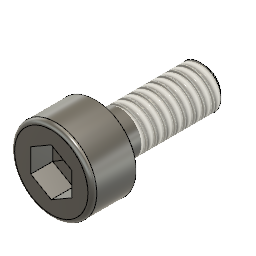
oscillating_design v15 (Autodesk Fusion 360 archive; units mm, degrees)
design "Broached Hexagon Socket Head Cap Screw ASME B18.3.1M - M1.6x0.35 x 4 Steel Grade 2 Plain"
description: Broached Hexagon Socket Head Cap Screw ASME B18.3.1M - M1.6x0.35 x 4
part number: BSHCS ASME B18.3.1M - M1.6x0.35 x 4 Steel Grade 2 Plain
Autodesk Fusion 360 part; units mm, degrees
sketch "Sketch1" plane through (0, 0, 0) normal (0, 1, 0) x (1, 0, 0)
  line L0 (-0.8, 0) -> (-0.8, 4)
  line L1 (-0.8, 4) -> (0, 4)
  line L2 (0, 4) -> (0, -1.6)
  line L3 (-0.8, 0) -> (-1.5, 0)
  line L4 (-1.5, 0) -> (-1.5, -1.6)
  line L5 (-1.5, -1.6) -> (0, -1.6)
  dimension "d9" = 1.6
  dimension "d66" = 3
  dimension "d101" = 4
  dimension "d102" = 1.6
  constraint perpendicular L0 L1
  constraint collinear origin L1.end L2.end
  constraint perpendicular L0 L3
  constraint coincident origin L3
  constraint vertical L0
  constraint vertical L2
  constraint parallel L2 L4
  constraint coincident L2 L5.end
  constraint perpendicular L2 L5
  measures "d101" distance of origin L1
  measures "d102" distance of L3.end L5
revolve "Revolve1" add sketch "Sketch1" angle 360 about axis through (0, 0, -4) along (0, 0, 1)
ref_plane "WorkPlane1" through (0, 0, 1.6) normal (0, 0, 1) x (1, 0, 0)
sketch "Sketch6" plane through (0, 0, 1.6) normal (0, 0, 1) x (1, 0, 0)
  line L0 (-0.75, 0) -> (0.75, 0) construction
  line L1 (0, 0) -> (-0.75, 0.433)
  line L2 (-0.75, -0.433) -> (-0.75, 0.433)
  line L3 (-0.75, -0.433) -> (0, 0)
  dimension "d100" = 150
  dimension "d103" = 1.5
  constraint horizontal L0
  constraint midpoint L1.start L0
  constraint coincident L1.start L3.end
  constraint perpendicular L0 L2
  constraint midpoint L0.start L2
  constraint coincident L1.end L2.end
  measures "d100" angle of L0 L1
  measures "d103" distance of L0.end L2
extrude "Extrude1" cut sketch "Sketch6" against normal blind 0.8
pattern_circular "C-Pattern1" count 6 over 360 about axis through (0, 0, 1.75) along (0, 0, 1) of "Extrude1"
extrude "Extrude2" cut 1 faces at (0, 0.2887, 0.8) along direction (0, 0, -1) blind 0.8 draft -85
thread "Thread2" "ANSI Metric M Profile 1.6 M1.6x0.35 4g6g" major diameter 1.5385 minor diameter 1.15 pitch 0.35 angle 60 resizes the face on face at (-0.796, 0.0797, -2.6667) from (0, 0, -0.9147) to (0, 0, -4)
fillet "Fillet4" radius 0.16 1 edges at (-1.3985, 0.5424, 1.6)
sketch "Sketch7" plane through (0, 0, 0) normal (0, 1, 0) x (1, 0, 0)
  line L0 (-0.816, 4) -> (-0.816, 3.7853)
  line L1 (-0.816, 3.7853) -> (-0.5853, 4)
  line L2 (0, 4) -> (0, -1.6)
  line L3 (-0.816, 4) -> (0, 4)
  dimension "d104" = 0.5853
  dimension "d105" = 0.816
  dimension "d106" = 0.2147
  constraint coincident L2.start L3.end
  constraint perpendicular L2 L3
  constraint coincident L1.end L3
  constraint perpendicular L0 L3
  measures "d104" distance of L1.end L2
  measures "d105" distance of L0 L2.start
  measures "d106" distance of L0.end L3
revolve "Revolve3" cut sketch "Sketch7" angle 360 about axis through (0, 0, 1.75) along (0, 0, 1)
equation "d9 = adsk_nomdia"
equation "adsk_nomlen = 4.00 mm"
equation "adsk_headh = 1.60 mm"
equation "adsk_headdia = 3.00 mm"
equation "adsk_nomdia = 1.60 mm"
equation "adsk_philwidth = 1.50 mm"
equation "d31 = -adsk_phildepth"
equation "adsk_phildepth = 0.80 mm"
equation "d66 = adsk_headdia"
equation "d71 = adsk_headh"
equation "d76 = -adsk_phildepth"
equation "adsk_thrlen = 3.0852925 mm"
equation "d84 = adsk_thrlen"
equation "d86 = adsk_nomdia * 0.1"
equation "adsk_startlen = 0.2147075 mm"
equation "adsk_endpointdia = 1.170585 mm"
equation "d101 = adsk_nomlen"
equation "d102 = adsk_headh"
equation "d103 = adsk_philwidth"
equation "d104 = adsk_endpointdia / 2"
equation "d105 = adsk_nomdia * 0.51"
equation "d106 = adsk_startlen"

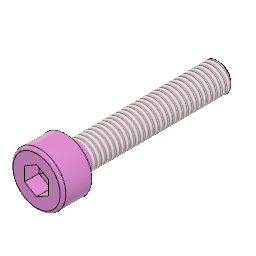
design "Broached Hexagon Socket Head Cap Screw ASME B18.3.1M - M3x0.5 x 16 Steel Grade 2 Plain"
description: Broached Hexagon Socket Head Cap Screw ASME B18.3.1M - M3x0.5 x 16
part number: BSHCS ASME B18.3.1M - M3x0.5 x 16 Steel Grade 2 Plain
Autodesk Fusion 360 part; units mm, degrees
sketch "Sketch1" plane through (0, 0, 0) normal (0, 1, 0) x (1, 0, 0)
  line L0 (-1.5, 0) -> (-1.5, 16)
  line L1 (-1.5, 16) -> (0, 16)
  line L2 (0, 16) -> (0, -3)
  line L3 (-1.5, 0) -> (-2.75, 0)
  line L4 (-2.75, 0) -> (-2.75, -3)
  line L5 (-2.75, -3) -> (0, -3)
  dimension "d9" = 3
  dimension "d66" = 5.5
  dimension "d101" = 16
  dimension "d102" = 3
  constraint perpendicular L0 L1
  constraint collinear origin L1.end L2.end
  constraint perpendicular L0 L3
  constraint coincident origin L3
  constraint vertical L0
  constraint vertical L2
  constraint parallel L2 L4
  constraint coincident L2 L5.end
  constraint perpendicular L2 L5
  measures "d101" distance of origin L1
  measures "d102" distance of L3.end L5
revolve "Revolve1" add sketch "Sketch1" angle 360 about axis through (0, 0, -16) along (0, 0, 1)
ref_plane "WorkPlane1" through (0, 0, 3) normal (0, 0, 1) x (1, 0, 0)
sketch "Sketch6" plane through (0, 0, 3) normal (0, 0, 1) x (1, 0, 0)
  line L0 (-1.25, 0) -> (1.25, 0) construction
  line L1 (0, 0) -> (-1.25, 0.7217)
  line L2 (-1.25, -0.7217) -> (-1.25, 0.7217)
  line L3 (-1.25, -0.7217) -> (0, 0)
  dimension "d100" = 150
  dimension "d103" = 2.5
  constraint horizontal L0
  constraint midpoint L1.start L0
  constraint coincident L1.start L3.end
  constraint perpendicular L0 L2
  constraint midpoint L0.start L2
  constraint coincident L1.end L2.end
  measures "d100" angle of L0 L1
  measures "d103" distance of L0.end L2
extrude "Extrude1" cut sketch "Sketch6" against normal blind 1.5
pattern_circular "C-Pattern1" count 6 over 360 about axis through (0, 0, 1.75) along (0, 0, 1) of "Extrude1"
extrude "Extrude2" cut 1 faces at (0, -0.4811, 1.5) along direction (0, 0, -1) blind 1.5 draft -85
thread "Thread2" "ANSI Metric M Profile 3.0 M3x0.5 4g6g" major diameter 2.927 minor diameter 2.369 pitch 0.5 angle 60 resizes the face on face at (-1.4925, 0.1494, -10.6667) from (0, 0, -1.3067) to (0, 0, -16)
fillet "Fillet4" radius 0.3 1 edges at (-2.5639, 0.9944, 3)
sketch "Sketch7" plane through (0, 0, 0) normal (0, 1, 0) x (1, 0, 0)
  line L0 (-1.53, 16) -> (-1.53, 15.6933)
  line L1 (-1.53, 15.6933) -> (-1.1933, 16)
  line L2 (0, 16) -> (0, -3)
  line L3 (-1.53, 16) -> (0, 16)
  dimension "d104" = 1.1933
  dimension "d105" = 1.53
  dimension "d106" = 0.3067
  constraint coincident L2.start L3.end
  constraint perpendicular L2 L3
  constraint coincident L1.end L3
  constraint perpendicular L0 L3
  measures "d104" distance of L1.end L2
  measures "d105" distance of L0 L2.start
  measures "d106" distance of L0.end L3
revolve "Revolve3" cut sketch "Sketch7" angle 360 about axis through (0, 0, 1.75) along (0, 0, 1)
equation "d9 = adsk_nomdia"
equation "adsk_nomlen = 16.00 mm"
equation "adsk_headh = 3.00 mm"
equation "adsk_headdia = 5.50 mm"
equation "adsk_nomdia = 3.00 mm"
equation "adsk_philwidth = 2.50 mm"
equation "d31 = -adsk_phildepth"
equation "adsk_phildepth = 1.50 mm"
equation "d66 = adsk_headdia"
equation "d71 = adsk_headh"
equation "d76 = -adsk_phildepth"
equation "adsk_thrlen = 14.693275 mm"
equation "d84 = adsk_thrlen"
equation "d86 = adsk_nomdia * 0.1"
equation "adsk_startlen = 0.306725 mm"
equation "adsk_endpointdia = 2.38655 mm"
equation "d101 = adsk_nomlen"
equation "d102 = adsk_headh"
equation "d103 = adsk_philwidth"
equation "d104 = adsk_endpointdia / 2"
equation "d105 = adsk_nomdia * 0.51"
equation "d106 = adsk_startlen"

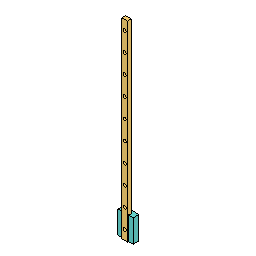
design "guide_rail"
Autodesk Fusion 360 part; units mm, degrees
sketch "Sketch1" plane through (0, 0, 0) normal (0, 1, 0) x (1, 0, 0)
  line L0 (0, 0) -> (8, 0)
  line L1 (8, 0) -> (8, -3)
  line L2 (8, -3) -> (5.5, -3)
  line L3 (0, 0) -> (0, -3)
  line L4 (0, -3) -> (2.5, -3)
  line L5 (2.5, -3) -> (2.5, -2)
  line L6 (2.5, -2) -> (5.5, -2)
  line L7 (5.5, -3) -> (5.5, -2)
  line L8 (2.5, -2) -> (2.5, -4)
  line L9 (2.5, -4) -> (5.5, -4)
  line L10 (5.5, -4) -> (5.5, -2)
  dimension "d1" = 8
  dimension "d2" = 3
  dimension "d3" = 2.5
  dimension "d4" = 3
  dimension "d5" = 2.5
  dimension "d6" = 1
  dimension "d7" = 2
  dimension "d8" = 3
  constraint coincident L0.start L3.start
  constraint horizontal L0
  constraint perpendicular L0 L1
  constraint perpendicular L1 L2
  constraint perpendicular L0 L3
  constraint perpendicular L3 L4
  constraint perpendicular L0 L5
  constraint perpendicular L5 L6
  constraint perpendicular L6 L7
  constraint perpendicular L6 L8
  constraint perpendicular L8 L9
  measures "d1" distance of L0.start L0.end
  measures "d2" distance of L0.end L1.end
  measures "d3" distance of L1.end L2.end
  measures "d4" distance of L0.start L3.end
  measures "d5" distance of L3.end L4.end
  measures "d6" distance of L4.end L5.end
  measures "d7" distance of L5.end L8.end
  measures "d8" distance of L8.end L9.end
extrude "Extrude1" add sketch "Sketch1" along normal mid plane 12 contours L0 L1 L2 L3 L4 L5 L6 L7 L8 L10 makes body 1
extrude "Extrude2" add sketch "Sketch1" along normal mid plane 100 separate body contours L5 L6 L7 L8 L9 L10 makes body 2
sketch "Sketch2" plane through (0, 0, 0) normal (0, 0, -1) x (-1, 0, 0)
  line L0 (0, -6) -> (0, 6)
  line L1 (0, 6) -> (-8, 6)
  line L2 (-8, 6) -> (-8, -6)
  line L3 (-8, -6) -> (0, -6)
  line L4 (-4, -6) -> (-4, 6)
  circle A0 centre (-4, -1.75) radius 0.8
  circle A1 centre (-4, 1.75) radius 0.8
  line L5 (-4, -0.95) -> (-4, 0.95) construction
  point P0 (-4, 0)
  dimension "d14" = 1.6
  dimension "d15" = 1.6
  dimension "d16" = 3.5
  constraint midpoint L3 L4.start
  constraint midpoint L1 L4.end
  constraint coincident L4 A0.centre
  constraint coincident L4 A1.centre
  constraint coincident L4 L5.start
  constraint coincident A0 L5.start
  constraint coincident L4 L5.end
  constraint coincident A1 L5.end
  constraint midpoint L5 P0
  measures "d14" diameter of A0
  measures "d15" diameter of A1
  measures "d16" distance of A0.centre A1.centre
extrude "Extrude3" cut sketch "Sketch2" against normal blind 1.3 contours L4 A0 | L4 A0 | L4 A1 | L4 A1 bodies 2 1
sketch "Sketch3" plane through (0, 0, 2) normal (0, 0, -1) x (-1, 0, 0)
  line L0 (-2.5, -50) -> (-2.5, 50)
  line L1 (-2.5, 50) -> (-5.5, 50)
  line L2 (-5.5, 50) -> (-5.5, -50)
  line L3 (-5.5, -50) -> (-2.5, -50)
  circle A0 centre (-4, -45) radius 0.8
  circle A1 centre (-4, -35) radius 0.8
  circle A2 centre (-4, -25) radius 0.8
  circle A3 centre (-4, -15) radius 0.8
  circle A4 centre (-4, -5) radius 0.8
  circle A5 centre (-4, 5) radius 0.8
  circle A6 centre (-4, 15) radius 0.8
  circle A7 centre (-4, 25) radius 0.8
  circle A8 centre (-4, 35) radius 0.8
  circle A9 centre (-4, 45) radius 0.8
  dimension "d19" = 1.6
  dimension "d20" = 5
  dimension "d38" = 0
  dimension "d39" = 10
  measures "d19" diameter of A0
  measures "d20" distance of L3 A0.centre
extrude "Extrude4" cut sketch "Sketch3" against normal blind 11.812 contours A0 | A1 | A2 | A3 | A4 | A5 | A6 | A7 | A8 | A9 bodies 2
copy_body "Body->Comp1" bodies 2 removing the originals makes body 3 in component "rail"
copy_body "Body->Comp2" bodies 1 removing the originals makes body 4 in component "cart"
component "rail" placed x (1, 0, 0) y (0, 1, 0) z (0, 0, 1) at (0, 0, 0)
component "cart" placed x (-1, 0, 0) y (0, -1, 0) z (0, 0, 1) at (8, -44, 0.5)
equation "rail_length = 100 mm"
equation "d12 = rail_length / 2"
named bodies: "cart", "rail"

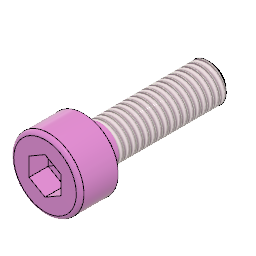
design "Broached Hexagon Socket Head Cap Screw ASME B18.3.1M - M3x0.5 x 10 Steel Grade 2 Plain"
description: Broached Hexagon Socket Head Cap Screw ASME B18.3.1M - M3x0.5 x 10
part number: BSHCS ASME B18.3.1M - M3x0.5 x 10 Steel Grade 2 Plain
Autodesk Fusion 360 part; units mm, degrees
sketch "Sketch1" plane through (0, 0, 0) normal (0, 1, 0) x (1, 0, 0)
  line L0 (-1.5, 0) -> (-1.5, 10)
  line L1 (-1.5, 10) -> (0, 10)
  line L2 (0, 10) -> (0, -3)
  line L3 (-1.5, 0) -> (-2.75, 0)
  line L4 (-2.75, 0) -> (-2.75, -3)
  line L5 (-2.75, -3) -> (0, -3)
  dimension "d9" = 3
  dimension "d66" = 5.5
  dimension "d101" = 10
  dimension "d102" = 3
  constraint perpendicular L0 L1
  constraint collinear origin L1.end L2.end
  constraint perpendicular L0 L3
  constraint coincident origin L3
  constraint vertical L0
  constraint vertical L2
  constraint parallel L2 L4
  constraint coincident L2 L5.end
  constraint perpendicular L2 L5
  measures "d101" distance of origin L1
  measures "d102" distance of L3.end L5
revolve "Revolve1" add sketch "Sketch1" angle 360 about axis through (0, 0, -10) along (0, 0, 1)
ref_plane "WorkPlane1" through (0, 0, 3) normal (0, 0, 1) x (1, 0, 0)
sketch "Sketch6" plane through (0, 0, 3) normal (0, 0, 1) x (1, 0, 0)
  line L0 (-1.25, 0) -> (1.25, 0) construction
  line L1 (0, 0) -> (-1.25, 0.7217)
  line L2 (-1.25, -0.7217) -> (-1.25, 0.7217)
  line L3 (-1.25, -0.7217) -> (0, 0)
  dimension "d100" = 150
  dimension "d103" = 2.5
  constraint horizontal L0
  constraint midpoint L1.start L0
  constraint coincident L1.start L3.end
  constraint perpendicular L0 L2
  constraint midpoint L0.start L2
  constraint coincident L1.end L2.end
  measures "d100" angle of L0 L1
  measures "d103" distance of L0.end L2
extrude "Extrude1" cut sketch "Sketch6" against normal blind 1.5
pattern_circular "C-Pattern1" count 6 over 360 about axis through (0, 0, 1.75) along (0, 0, 1) of "Extrude1"
extrude "Extrude2" cut 1 faces at (0, -0.4811, 1.5) along direction (0, 0, -1) blind 1.5 draft -85
thread "Thread2" "ANSI Metric M Profile 3.0 M3x0.5 4g6g" major diameter 2.927 minor diameter 2.369 pitch 0.5 angle 60 resizes the face on face at (-1.4925, 0.1494, -6.6667) from (0, 0, -1.3067) to (0, 0, -10)
fillet "Fillet4" radius 0.3 1 edges at (-2.5639, 0.9944, 3)
sketch "Sketch7" plane through (0, 0, 0) normal (0, 1, 0) x (1, 0, 0)
  line L0 (-1.53, 10) -> (-1.53, 9.6933)
  line L1 (-1.53, 9.6933) -> (-1.1933, 10)
  line L2 (0, 10) -> (0, -3)
  line L3 (-1.53, 10) -> (0, 10)
  dimension "d104" = 1.1933
  dimension "d105" = 1.53
  dimension "d106" = 0.3067
  constraint coincident L2.start L3.end
  constraint perpendicular L2 L3
  constraint coincident L1.end L3
  constraint perpendicular L0 L3
  measures "d104" distance of L1.end L2
  measures "d105" distance of L0 L2.start
  measures "d106" distance of L0.end L3
revolve "Revolve3" cut sketch "Sketch7" angle 360 about axis through (0, 0, 1.75) along (0, 0, 1)
equation "d9 = adsk_nomdia"
equation "adsk_nomlen = 10.00 mm"
equation "adsk_headh = 3.00 mm"
equation "adsk_headdia = 5.50 mm"
equation "adsk_nomdia = 3.00 mm"
equation "adsk_philwidth = 2.50 mm"
equation "d31 = -adsk_phildepth"
equation "adsk_phildepth = 1.50 mm"
equation "d66 = adsk_headdia"
equation "d71 = adsk_headh"
equation "d76 = -adsk_phildepth"
equation "adsk_thrlen = 8.693275 mm"
equation "d84 = adsk_thrlen"
equation "d86 = adsk_nomdia * 0.1"
equation "adsk_startlen = 0.306725 mm"
equation "adsk_endpointdia = 2.38655 mm"
equation "d101 = adsk_nomlen"
equation "d102 = adsk_headh"
equation "d103 = adsk_philwidth"
equation "d104 = adsk_endpointdia / 2"
equation "d105 = adsk_nomdia * 0.51"
equation "d106 = adsk_startlen"

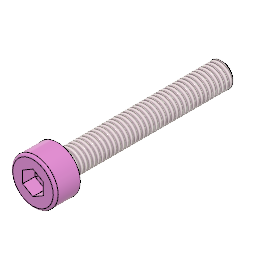
design "Broached Hexagon Socket Head Cap Screw ASME B18.3.1M - M3x0.5 x 20 Steel Grade 2 Plain"
description: Broached Hexagon Socket Head Cap Screw ASME B18.3.1M - M3x0.5 x 20
part number: BSHCS ASME B18.3.1M - M3x0.5 x 20 Steel Grade 2 Plain
Autodesk Fusion 360 part; units mm, degrees
sketch "Sketch1" plane through (0, 0, 0) normal (0, 1, 0) x (1, 0, 0)
  line L0 (-1.5, 0) -> (-1.5, 20)
  line L1 (-1.5, 20) -> (0, 20)
  line L2 (0, 20) -> (0, -3)
  line L3 (-1.5, 0) -> (-2.75, 0)
  line L4 (-2.75, 0) -> (-2.75, -3)
  line L5 (-2.75, -3) -> (0, -3)
  dimension "d9" = 3
  dimension "d66" = 5.5
  dimension "d101" = 20
  dimension "d102" = 3
  constraint perpendicular L0 L1
  constraint collinear origin L1.end L2.end
  constraint perpendicular L0 L3
  constraint coincident origin L3
  constraint vertical L0
  constraint vertical L2
  constraint parallel L2 L4
  constraint coincident L2 L5.end
  constraint perpendicular L2 L5
  measures "d101" distance of origin L1
  measures "d102" distance of L3.end L5
revolve "Revolve1" add sketch "Sketch1" angle 360 about axis through (0, 0, -20) along (0, 0, 1)
ref_plane "WorkPlane1" through (0, 0, 3) normal (0, 0, 1) x (1, 0, 0)
sketch "Sketch6" plane through (0, 0, 3) normal (0, 0, 1) x (1, 0, 0)
  line L0 (-1.25, 0) -> (1.25, 0) construction
  line L1 (0, 0) -> (-1.25, 0.7217)
  line L2 (-1.25, -0.7217) -> (-1.25, 0.7217)
  line L3 (-1.25, -0.7217) -> (0, 0)
  dimension "d100" = 150
  dimension "d103" = 2.5
  constraint horizontal L0
  constraint midpoint L1.start L0
  constraint coincident L1.start L3.end
  constraint perpendicular L0 L2
  constraint midpoint L0.start L2
  constraint coincident L1.end L2.end
  measures "d100" angle of L0 L1
  measures "d103" distance of L0.end L2
extrude "Extrude1" cut sketch "Sketch6" against normal blind 1.5
pattern_circular "C-Pattern1" count 6 over 360 about axis through (0, 0, 1.75) along (0, 0, 1) of "Extrude1"
extrude "Extrude2" cut 1 faces at (0, -0.4811, 1.5) along direction (0, 0, -1) blind 1.5 draft -85
thread "Thread2" "ANSI Metric M Profile 3.0 M3x0.5 4g6g" major diameter 2.927 minor diameter 2.369 pitch 0.5 angle 60 resizes the face on face at (-1.4925, 0.1494, -13.3333) from (0, 0, -0.9135) to (0, 0, -20)
fillet "Fillet4" radius 0.3 1 edges at (-2.5639, 0.9944, 3)
sketch "Sketch7" plane through (0, 0, 0) normal (0, 1, 0) x (1, 0, 0)
  line L0 (-1.53, 20) -> (-1.53, 19.6933)
  line L1 (-1.53, 19.6933) -> (-1.1933, 20)
  line L2 (0, 20) -> (0, -3)
  line L3 (-1.53, 20) -> (0, 20)
  dimension "d104" = 1.1933
  dimension "d105" = 1.53
  dimension "d106" = 0.3067
  constraint coincident L2.start L3.end
  constraint perpendicular L2 L3
  constraint coincident L1.end L3
  constraint perpendicular L0 L3
  measures "d104" distance of L1.end L2
  measures "d105" distance of L0 L2.start
  measures "d106" distance of L0.end L3
revolve "Revolve3" cut sketch "Sketch7" angle 360 about axis through (0, 0, 1.75) along (0, 0, 1)
equation "d9 = adsk_nomdia"
equation "adsk_nomlen = 20.00 mm"
equation "adsk_headh = 3.00 mm"
equation "adsk_headdia = 5.50 mm"
equation "adsk_nomdia = 3.00 mm"
equation "adsk_philwidth = 2.50 mm"
equation "d31 = -adsk_phildepth"
equation "adsk_phildepth = 1.50 mm"
equation "d66 = adsk_headdia"
equation "d71 = adsk_headh"
equation "d76 = -adsk_phildepth"
equation "adsk_thrlen = 19.08655 mm"
equation "d84 = adsk_thrlen"
equation "d86 = adsk_nomdia * 0.1"
equation "adsk_startlen = 0.306725 mm"
equation "adsk_endpointdia = 2.38655 mm"
equation "d101 = adsk_nomlen"
equation "d102 = adsk_headh"
equation "d103 = adsk_philwidth"
equation "d104 = adsk_endpointdia / 2"
equation "d105 = adsk_nomdia * 0.51"
equation "d106 = adsk_startlen"

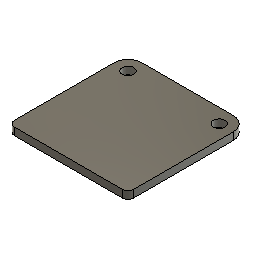
design "laser"
Autodesk Fusion 360 part; units mm, degrees
sketch "Sketch1" plane through (0, 0, 0) normal (0, 1, 0) x (1, 0, 0)
  line L0 (3, 0) -> (22.4, 0)
  line L1 (25.4, -3) -> (25.4, -24.13)
  line L2 (24.13, -25.4) -> (1.27, -25.4)
  line L3 (0, -24.13) -> (0, -3)
  line L4 (12.7, 0) -> (12.7, -25.4)
  circle A0 centre (3, -3) radius 1.25
  circle A1 centre (22.4, -3) radius 1.25
  arc A2 (3, 0) -> (0, -3) centre (3, -3) ccw
  arc A3 (25.4, -3) -> (22.4, 0) centre (22.4, -3) ccw
  arc A4 (0, -24.13) -> (1.27, -25.4) centre (1.27, -24.13) ccw
  arc A5 (24.13, -25.4) -> (25.4, -24.13) centre (24.13, -24.13) ccw
  point P0 (25.4, 0)
  point P1 (0, -25.4)
  dimension "d1" = 25.4
  dimension "d2" = 25.4
  dimension "d3" = 2.5
  dimension "d4" = 22.4
  dimension "d5" = 19.4
  dimension "d6" = 3
  dimension "d7" = 1.27
  constraint horizontal L0
  constraint vertical L1
  constraint horizontal L2
  constraint vertical L3
  constraint symmetric L4 A0 A1
  constraint coincident L0 L4.start
  constraint coincident origin L0
  constraint coincident origin L3
  constraint tangent L0 A2
  constraint tangent L3 A2
  constraint coincident P0 L0
  constraint coincident P0 L1
  constraint tangent L0 A3
  constraint tangent L1 A3
  constraint equal A2 A3
  constraint coincident L2 L4.end
  constraint coincident P1 L2
  constraint coincident P1 L3
  constraint tangent L2 A4
  constraint tangent L3 A4
  constraint tangent L1 A5
  constraint tangent L2 A5
  constraint equal A4 A5
  measures "d1" distance of origin P0
  measures "d2" distance of origin P1
  measures "d3" diameter of A0
  measures "d4" distance of L2 A0.centre
  measures "d5" distance of A0.centre A1.centre
  measures "d6" radius of A2
  measures "d7" radius of A4
extrude "Extrude1" add sketch "Sketch1" along normal blind 1.6
